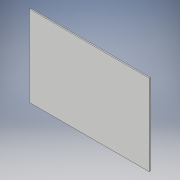
# Autodesk Inventor part: Pièce-interieur-3
Saved by Autodesk Inventor 2019 (Build 230136000, 136)
## iProperties
Created: 2018-12-30
Part Number: Pièce-interieur-3
Material: Générique
Document SubType Name: Modeling
Designer: pouey
Density: 1 g/cm^3
Appearance: Par défaut
Author: pouey
Autodesk Inventor part; units mm, degrees
ref_plane "YZ Plane" through (0, 0, 0) normal (1, 0, 0) x (0, 1, 0)
ref_plane "XZ Plane" through (0, 0, 0) normal (0, 1, 0) x (-1, 0, 0)
ref_plane "XY Plane" through (0, 0, 0) normal (0, 0, 1) x (1, 0, 0)
sketch "Esquisse1" plane through (0, 0, 0) normal (0, 0, 1) x (1, 0, 0)
  line L0 (0, 0) -> (295, 0)
  line L1 (295, 0) -> (295, 200)
  line L2 (295, 200) -> (0, 200)
  line L3 (0, 200) -> (0, 0)
  dimension "d0" = 295
  dimension "d1" = 200
  constraints: 8 end point, 2 parallel, 1 horizontal, 1 perpendicular
  measures "d0" distance of L1.end L2.end
  measures "d1" distance of L0.end L1.end
extrude "Extrusion1" add sketch "Esquisse1" along normal blind 3
